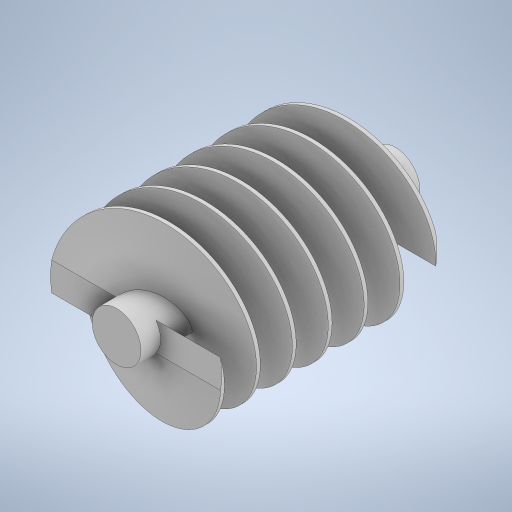
# Autodesk Inventor part: spiral
Saved by Autodesk Inventor 2023 (Build 270158000, 158)
## iProperties
Created: 2023-02-17
Part Number: spiral
Material: Generic
Document SubType Name: Modeling
Designer: caleb
Density: 1 g/cm^3
Appearance: Default
Author: caleb
## iProperties of the stored document spiral_3DPrint.ipt
Created: 2023-02-28
Part Number: spiral_3DPrint
Material: Generic
Document SubType Name: Modeling
Designer: caleb
Density: 1 g/cm^3
Appearance: Default
Author: caleb
Autodesk Inventor part; units mm, degrees
ref_plane "YZ Plane" through (0, 0, 0) normal (1, 0, 0) x (0, 1, 0)
ref_plane "XZ Plane" through (0, 0, 0) normal (0, 1, 0) x (-1, 0, 0)
ref_plane "XY Plane" through (0, 0, 0) normal (0, 0, 1) x (1, 0, 0)
sketch "Sketch1" plane through (0, 0, 0) normal (0, 0, 1) x (1, 0, 0)
  circle A0 centre (0, 0) radius 17.5
  circle A1 centre (0, 0) radius 5
  line L0 (-17.2552, 2.9167) -> (17.2552, 2.9167)
  line L1 (17.2552, -2.9167) -> (-17.2552, -2.9167)
  point P0 (-4.0612, -2.9167)
  point P1 (-4.0612, 2.9167)
  point P2 (4.0612, -2.9167)
  point P3 (4.0612, 2.9167)
  dimension "d0" = 35
  dimension "d1" = 10
  constraints: 4 end point, 4 point on circle, 2 centre point, 2 coincident, 1 horizontal, 1 parallel
  measures "d0" diameter of A0
  measures "d1" diameter of A1
extrude "Extrusion1" add sketch "Sketch1" against normal blind 44 contours L0 A1 | A1 L1 L0 | A1 L1
sketch "Sketch2" plane through (0, 0, -44) normal (0, 0, -1) x (-1, 0, 0)
  circle A0 centre (0, 0) radius 17.5 projected
  line L0 (17.2552, 2.9167) -> (-17.2552, 2.9167) projected
  line L1 (-17.2552, -2.9167) -> (17.2552, -2.9167) projected
  circle A1 centre (0, 0) radius 5 projected
  line L2 (-1.25, 1.25) -> (1.25, 1.25)
  line L3 (1.25, 1.25) -> (1.25, -1.25)
  line L4 (1.25, -1.25) -> (-1.25, -1.25)
  line L5 (-1.25, -1.25) -> (-1.25, 1.25)
  line L6 (-1.25, 1.25) -> (1.25, -1.25) construction
  line L7 (1.25, 1.25) -> (-1.25, -1.25) construction
  dimension "d12" = 2.5
  dimension "d13" = 2.5
  constraints: 12 end point, 2 midpoint, 2 parallel, 1 horizontal, 1 perpendicular
  measures "d12" distance of L3.end L4.end
  measures "d13" distance of L2.end L3.end
sketch3d "3D Sketch1"
  helix H0 starts at (-7.3951, 1.25, 0) axis through (0, 0, 0) along (0, 0, -1) pitch 14.6667 turns 3 hand right
sweep "Sweep1" add profiles "Sketch1" path "3D Sketch1" contours A0 L1 A1 L0 | L0 A1 L1 A0
extrude "Extrusion3" cut sketch "Sketch2" against normal blind 15 contours L2 L3 L4 L5
extrude "Extrusion4" add sketch "Sketch1" along normal blind 4 contours L0 A1 | A1 L1 L0 | A1 L1
extrude "Extrusion5" add sketch "Sketch2" along normal blind 9 contours A1 L1 L0 | L0 A1 | A1 L1
body "Solid1"
